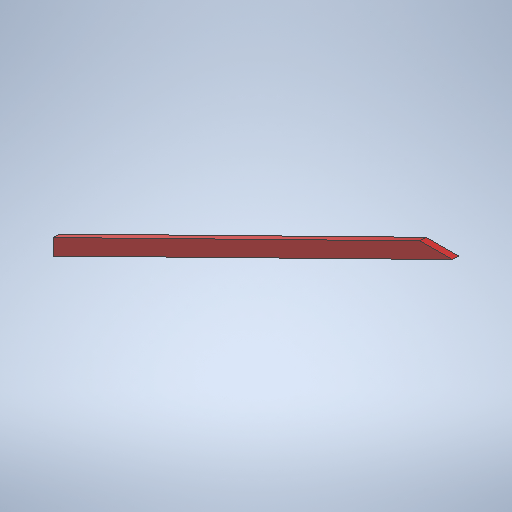
# Autodesk Inventor part: s48'x2x4
Saved by Autodesk Inventor 2025.1 (Build 291241020, 241B)
## iProperties
Created: 2024-09-16
Part Number: s48'x2x4
Material: Generic
Document SubType Name: Modeling
Designer: User
Density: 1 g/cm^3
Appearance: Default
Author: User
Autodesk Inventor part; units mm, degrees
ref_plane "YZ Plane" through (0, 0, 0) normal (1, 0, 0) x (0, 1, 0)
ref_plane "XZ Plane" through (0, 0, 0) normal (0, 1, 0) x (-1, 0, 0)
ref_plane "XY Plane" through (0, 0, 0) normal (0, 0, 1) x (1, 0, 0)
sketch "Sketch1" plane through (0, 0, 0) normal (0, 0, 1) x (1, 0, 0)
  line L0 (0, 3619.5) -> (0, -1257.3) projected
  line L1 (0, -38.1) -> (2438.4, -38.1) projected
  line L2 (2476.5, -38.1) -> (2438.4, -38.1) projected
  line L3 (2476.5, -38.1) -> (0, -1257.3)
  line L4 (0, -1158.2107) -> (2275.2249, -38.1)
  line L5 (2275.2249, -38.1) -> (2476.5, -38.1)
  line L6 (0, -1257.3) -> (0, -1158.2107)
  point P0 (0, 0)
  dimension "d0" = 88.9
  constraints: 8 end point, 2 collinear, 2 point on line, 1 parallel, 3 other
  measures "d0" distance between parallel lines of L4 L3
extrude "Extrusion1" add sketch "Sketch1" against normal blind 38.1 contours L4 L1 L2 L3 L0
body "Solid1"
